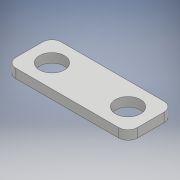
# Autodesk Inventor part: WeldAntiWarp
Saved by Autodesk Inventor 2018 (Build 220112000, 112)
## iProperties
Created: 2018-06-23
Part Number: WeldAntiWarp
Material: Generic
Document SubType Name: Modeling
Designer: eroldan
Density: 1 g/cm^3
Appearance: Default
Author: eroldan
Autodesk Inventor part; units mm, degrees
ref_plane "YZ Plane" through (0, 0, 0) normal (1, 0, 0) x (0, 1, 0)
ref_plane "XZ Plane" through (0, 0, 0) normal (0, 1, 0) x (-1, 0, 0)
ref_plane "XY Plane" through (0, 0, 0) normal (0, 0, 1) x (1, 0, 0)
sketch "Sketch1" plane through (0, 0, 0) normal (0, 0, 1) x (1, 0, 0)
  line L0 (-22.5, 0) -> (22.5, 0) construction
  circle A0 centre (33.5, 0) radius 11
  line L1 (-53.5, -20) -> (53.5, -20)
  line L2 (53.5, -20) -> (53.5, 20)
  line L3 (53.5, 20) -> (-53.5, 20)
  line L4 (-53.5, 20) -> (-53.5, -20)
  line L5 (-53.5, -20) -> (53.5, 20) construction
  line L6 (53.5, -20) -> (-53.5, 20) construction
  point P0 (0, 0)
  point P1 (0, 0)
  dimension "d4" = 22
  dimension "d3" = 45
  dimension "d11" = 20
  dimension "d12" = 20
  constraints: 14 end point, 3 midpoint, 2 horizontal, 2 horizontal alignment, 2 parallel, 1 coincident, 1 perpendicular, 2 other
  measures "d3" distance of L0.start L0.end
  measures "d11" distance from line of L2 point (33.5, 0)
  measures "d12" distance from line of L1 point (33.5, 0)
extrude "Extrusion1" add sketch "Sketch1" against normal blind 8 contours A0 | L4 L3 L2 L1
extrude "Extrusion2" cut sketch "Sketch1" against normal through all contours A0
mirror "Mirror1" about plane through (0, 0, 0) normal (1, 0, 0) of "Extrusion2"
fillet "Fillet1" radius 8.25 4 edges at (-53.5, 20, -4) (53.5, 20, -4) (53.5, -20, -4) (-53.5, -20, -4)
body "Solid1"
